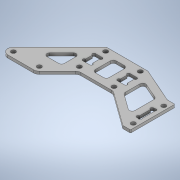
# Autodesk Inventor part: Head_side_frame_
Saved by Autodesk Inventor 2020.4 (Build 244396000, 396)
## iProperties
Created: 2022-01-01
Part Number: Head_side_frame_
Material: GFRP
Document SubType Name: Modeling
Designer: Masato Kubotera
Density: 1.75 g/cm^3
Appearance: 滑らか - 標準の灰色
Description: GFRP T2
Mass: 6.0022 g
Surface Area: 45.99 cm^2
Volume: 3.42983 cm^3
Author: Masato Kubotera
Autodesk Inventor part; units mm, degrees
ref_plane "YZ Plane" through (0, 0, 0) normal (1, 0, 0) x (0, 1, 0)
ref_plane "XZ Plane" through (0, 0, 0) normal (0, 1, 0) x (-1, 0, 0)
ref_plane "XY Plane" through (0, 0, 0) normal (0, 0, 1) x (1, 0, 0)
derived "Head_basis.ipt"
sketch "スケッチ1" plane through (0, 0, 0) normal (0, 1, 0) x (-1, 0, 0)
  line L0 (-44.985, 63.28) -> (-70.7944, 37.4706) construction
  line L1 (5.295, 20.5) -> (-9.705, 20.5)
  line L2 (-2.205, 20.5) -> (-44.985, 63.28) construction
  line L3 (-2.205, 20.5) -> (-2.205, 4.9887) construction
  line L4 (-54.1774, 43.481) -> (-57.7129, 47.0165) construction
  line L5 (-57.7129, 47.0165) -> (-80.3403, 24.3891) construction
  line L6 (-80.3403, 24.3891) -> (-76.8048, 20.8536) construction
  line L7 (-76.8048, 20.8536) -> (-54.1774, 43.481) construction
  line L8 (-54.1774, 43.481) -> (-80.3403, 24.3891) construction
  line L9 (-57.7129, 47.0165) -> (-76.8048, 20.8536) construction
  line L10 (-61.9555, 39.2383) -> (-72.5621, 28.6317) construction
  line L11 (-70.7944, 26.864) -> (-60.1878, 37.4706) construction
  circle A0 centre (-59.4807, 41.7132) radius 1.6
  line L12 (-55.9451, 45.2487) -> (-78.5725, 22.6213) construction
  line L13 (7.845, -2.5) -> (7.845, 2.5) construction
  line L14 (17.795, -2.5) -> (-22.205, -2.5) construction
  line L15 (6.3601, -2.5) -> (6.3601, 2.5) construction
  line L16 (7.795, -2.5) -> (7.795, 2.5)
  line L17 (11.414, 2.5) -> (7.545, 2.5)
  line L18 (-12.205, -2.5) -> (-12.205, 2.5)
  line L19 (5.6411, 2.5) -> (7.6411, 2.5)
  line L20 (-17.705, 0.5) -> (-15.205, 0.5)
  line L21 (7.795, 2.5) -> (-12.205, 2.5)
  line L22 (-15.205, 2.5) -> (10.795, 2.5) construction
  line L23 (-24.705, -2.5) -> (20.295, -2.5)
  arc A1 (7.795, -2.5) -> (9.895, -2.5) centre (8.845, -2.5) ccw
  line L24 (9.795, -2.5) -> (11.795, -2.5)
  line L25 (9.795, -2.5) -> (22.795, -2.5)
  line L26 (22.795, -2.5) -> (22.795, -5.5)
  line L27 (22.795, -5.5) -> (14.045, -5.5)
  line L28 (17.795, -2.5) -> (17.795, -5.5) construction
  arc A2 (-14.305, -2.5) -> (-12.205, -2.5) centre (-13.255, -2.5) ccw
  line L29 (-14.205, -2.5) -> (-27.205, -2.5)
  line L30 (-27.205, -2.5) -> (-27.205, -5.5)
  line L31 (-22.205, -2.5) -> (-22.205, -5.5) construction
  line L32 (-18.455, -5.5) -> (-27.205, -5.5)
  circle A3 centre (-11.5482, -8.5) radius 2
  arc A4 (14.045, -5.5) -> (11.1379, -8.4177) centre (14.045, -8.4071) ccw
  line L33 (15.045, -5.5) -> (15.045, -6.9) construction
  line L34 (15.045, -6.9) -> (20.545, -6.9) construction
  line L35 (20.545, -5.5) -> (20.545, -6.9) construction
  circle A5 centre (-11.5482, -8.5) radius 4
  line L36 (22.795, -2.5) -> (22.795, 0.5)
  line L37 (-2.205, -12.0113) -> (-2.205, 4.9887) construction
  line L38 (-19.455, -5.5) -> (-19.455, -6.9) construction
  line L39 (-19.455, -6.9) -> (-24.955, -6.9) construction
  line L40 (-24.955, -5.5) -> (-24.955, -6.9) construction
  line L41 (-69.0266, 35.7028) -> (-65.4911, 32.1673) construction
  circle A6 centre (-75.037, 26.1569) radius 1.6
  line L42 (-32.205, -2.5) -> (-22.205, -2.5)
  circle A7 centre (1.665, -21.7132) radius 2
  arc A8 (4.4934, -24.5416) -> (11.1379, -8.4177) centre (-11.5482, -8.5) ccw
  line L43 (-14.3767, -11.3284) -> (-1.1635, -24.5416)
  circle A9 centre (1.665, -21.7132) radius 4
  line L44 (4.4934, -18.8848) -> (-8.7198, -5.6716)
  line L45 (1.665, -21.7132) -> (-11.5482, -8.5) construction
  line L46 (-49.2969, -22.1777) -> (-31.6192, -4.5) construction
  line L47 (-31.6192, -4.5) -> (-28.0837, -8.0355) construction
  line L48 (-28.0837, -8.0355) -> (-45.7614, -25.7132) construction
  line L49 (-45.7614, -25.7132) -> (-49.2969, -22.1777) construction
  line L50 (-49.2969, -22.1777) -> (-28.0837, -8.0355) construction
  line L51 (-31.6192, -4.5) -> (-45.7614, -25.7132) construction
  line L52 (-47.5291, -23.9454) -> (-29.8515, -6.2678) construction
  line L53 (-40.4581, -13.3388) -> (-36.9225, -16.8744) construction
  line L54 (-40.1045, -20.0563) -> (-33.7405, -13.6924) construction
  line L55 (-33.7405, -13.6924) -> (-37.2761, -10.1569) construction
  line L56 (-37.2761, -10.1569) -> (-43.64, -16.5208) construction
  line L57 (-43.64, -16.5208) -> (-40.1045, -20.0563) construction
  line L58 (-40.1045, -20.0563) -> (-37.2761, -10.1569) construction
  line L59 (-33.7405, -13.6924) -> (-43.64, -16.5208) construction
  circle A10 centre (-45.4078, -21.8241) radius 1.6
  line L60 (-42.2258, -15.0359) -> (-38.761, -11.5711)
  line L61 (-37.2761, -10.0861) -> (-33.6698, -13.6924)
  line L62 (-35.1548, -15.1773) -> (-38.6196, -18.6421)
  line L63 (-40.1045, -20.1271) -> (-43.7107, -16.5208)
  line L64 (-43.7107, -16.5208) -> (-33.6698, -13.6924) construction
  line L65 (-37.2761, -10.0861) -> (-40.1045, -20.1271) construction
  arc A11 (-42.2258, -15.0359) -> (-43.7107, -16.5208) centre (-42.9683, -15.7784) ccw
  arc A12 (-37.2761, -10.0861) -> (-38.761, -11.5711) centre (-38.0185, -10.8286) ccw
  circle A13 centre (-31.9728, -8.3891) radius 1.6
  line L66 (-41.8723, -18.2886) -> (-35.5083, -11.9246) construction
  arc A14 (-40.1045, -20.1271) -> (-38.6196, -18.6421) centre (-39.362, -19.3846) ccw
  arc A15 (-35.1548, -15.1773) -> (-33.6698, -13.6924) centre (-34.4123, -14.4349) ccw
  line L67 (-32.205, 14.5) -> (-24.205, 22.5)
  circle A16 centre (-32.205, -2.5) radius 1 construction
  line L68 (-11.5482, -4.5) -> (-31.6192, -4.5)
  line L69 (-58.0664, 47.3701) -> (-54.1774, 43.481)
  line L70 (-76.8048, 20.8536) -> (-80.6939, 24.7426)
  line L71 (-80.6939, 24.7426) -> (-58.0664, 47.3701)
  line L72 (-45.7614, -25.7132) -> (1.665, -25.7132)
  line L73 (-45.7614, -25.7132) -> (-49.2969, -22.1777)
  arc A17 (-15.5479, -8.4464) -> (-18.455, -5.5) centre (-18.455, -8.4074) ccw
  line L74 (-49.2969, 13.1777) -> (-45.7614, 9.6421) construction
  line L75 (-45.7614, 9.6421) -> (-63.439, -8.0355) construction
  line L76 (-49.2969, 13.1777) -> (-63.439, -8.0355) construction
  arc A18 (-59.9035, 2.6418) -> (-61.3884, 1.1569) centre (-60.646, 1.8993) ccw
  line L77 (-52.8324, 2.5004) -> (-56.2972, -0.9645)
  line L78 (-57.7822, -2.4494) -> (-61.3884, 1.1569)
  line L79 (-61.3177, 1.1569) -> (-57.7822, -2.3787) construction
  line L80 (-66.9746, -4.5) -> (-49.2969, 13.1777) construction
  line L81 (-58.1357, 4.3388) -> (-54.6002, 0.8033) construction
  arc A19 (-57.7822, -2.4494) -> (-56.2972, -0.9645) centre (-57.0397, -1.7069) ccw
  line L82 (-59.5499, -0.6109) -> (-53.186, 5.753) construction
  line L83 (-59.9035, 2.6418) -> (-56.4387, 6.1066)
  line L84 (-51.4182, 3.9853) -> (-61.3177, 1.1569) construction
  line L85 (-61.3884, 1.1569) -> (-51.3475, 3.9853) construction
  arc A20 (-52.8324, 2.5004) -> (-51.3475, 3.9853) centre (-52.09, 3.2428) ccw
  line L86 (-57.7822, -2.3787) -> (-51.4182, 3.9853) construction
  line L87 (-54.9537, 7.5208) -> (-61.3177, 1.1569) construction
  arc A21 (-54.9537, 7.5915) -> (-56.4387, 6.1066) centre (-55.6962, 6.8491) ccw
  line L88 (-57.7822, -2.3787) -> (-54.9537, 7.5208) construction
  line L89 (-51.4182, 3.9853) -> (-54.9537, 7.5208) construction
  line L90 (-54.9537, 7.5915) -> (-51.3475, 3.9853)
  circle A22 centre (-49.6504, 9.2886) radius 1.6
  line L91 (-66.9746, -4.5) -> (-45.7614, 9.6421) construction
  line L92 (-65.2068, -6.2678) -> (-47.5291, 11.4099) construction
  line L93 (-54.9537, 7.5915) -> (-57.7822, -2.4494) construction
  line L94 (-63.439, -8.0355) -> (-66.9746, -4.5) construction
  circle A23 centre (-63.0855, -4.1464) radius 1.6
  line L95 (-63.439, -8.0355) -> (-66.9746, -4.5)
  line L96 (-31.6192, -4.5) -> (-45.7614, 9.6421)
  line L97 (-49.2969, 13.1777) -> (-45.7614, 9.6421)
  line L98 (-49.2969, 13.1777) -> (-54.1774, 43.481)
  line L99 (-76.8048, 20.8536) -> (-66.9746, -4.5)
  line L100 (-63.439, -8.0355) -> (-49.2969, -22.1777)
  line L101 (-54.1774, 43.481) -> (-76.8048, 20.8536) construction
  line L102 (-56.9363, 29.166) -> (-54.8022, 15.9153)
  line L103 (-55.3626, 14.1831) -> (-62.9161, 6.6295)
  line L104 (-66.1951, 7.3207) -> (-70.4935, 18.407)
  line L105 (-70.043, 20.5443) -> (-60.3251, 30.2622)
  arc A24 (-56.9363, 29.166) -> (-60.3251, 30.2622) centre (-58.9109, 28.848) ccw
  arc A25 (-70.043, 20.5443) -> (-70.4935, 18.407) centre (-68.6288, 19.13) ccw
  arc A26 (-66.1951, 7.3207) -> (-62.9161, 6.6295) centre (-64.3303, 8.0437) ccw
  arc A27 (-55.3626, 14.1831) -> (-54.8022, 15.9153) centre (-56.7768, 15.5973) ccw
  line L106 (-15.4772, -17.299) -> (-21.4624, -11.3138)
  line L107 (-24.2908, -11.3138) -> (-30.2761, -17.299)
  line L108 (-28.8619, -20.7132) -> (-16.8914, -20.7132)
  arc A28 (-16.8914, -20.7132) -> (-15.4772, -17.299) centre (-16.8914, -18.7132) ccw
  arc A29 (-21.4624, -11.3138) -> (-24.2908, -11.3138) centre (-22.8766, -12.728) ccw
  arc A30 (-30.2761, -17.299) -> (-28.8619, -20.7132) centre (-28.8619, -18.7132) ccw
  line L109 (-40.1045, -3.0858) -> (-44.3471, 1.1569)
  line L110 (-47.1756, 1.1569) -> (-54.9537, -6.6213)
  line L111 (-54.9537, -9.4497) -> (-50.7111, -13.6924)
  line L112 (-47.8827, -13.6924) -> (-40.1045, -5.9142)
  arc A31 (-40.1045, -5.9142) -> (-40.1045, -3.0858) centre (-41.5187, -4.5) ccw
  arc A32 (-44.3471, 1.1569) -> (-47.1756, 1.1569) centre (-45.7614, -0.2574) ccw
  arc A33 (-54.9537, -6.6213) -> (-54.9537, -9.4497) centre (-53.5395, -8.0355) ccw
  arc A34 (-50.7111, -13.6924) -> (-47.8827, -13.6924) centre (-49.2969, -12.2782) ccw
  circle A35 centre (-11.5482, -8.5) radius 1.6
  circle A36 centre (1.665, -21.7132) radius 1.6
  line L113 (-61.2484, 36.4099) -> (-69.7337, 27.9246) construction
  line L114 (-69.7337, 27.9246) -> (-71.5015, 29.6924) construction
  line L115 (-71.5015, 29.6924) -> (-63.0162, 38.1777) construction
  line L116 (-63.0162, 38.1777) -> (-61.2484, 36.4099) construction
  line L117 (-61.2484, 36.4099) -> (-71.5015, 29.6924) construction
  line L118 (-69.7337, 27.9246) -> (-63.0162, 38.1777) construction
  line L119 (-62.1323, 37.2938) -> (-70.6176, 28.8085) construction
  line L120 (-61.1777, 36.4099) -> (-63.0162, 38.2484)
  line L121 (-63.0162, 38.2484) -> (-71.5722, 29.6924)
  line L122 (-71.5722, 29.6924) -> (-69.7337, 27.8539)
  line L123 (-69.7337, 27.8539) -> (-61.1777, 36.4099)
  line L124 (-61.1777, 36.4099) -> (-71.5722, 29.6924) construction
  line L125 (-63.0162, 38.2484) -> (-69.7337, 27.8539) construction
  arc A37 (-62.6626, 34.925) -> (-61.1777, 36.4099) centre (-61.9202, 35.6674) ccw
  arc A38 (-61.9662, 37.1984) -> (-64.0662, 37.1984) centre (-63.0162, 37.1984) ccw
  arc A39 (-69.7337, 27.8539) -> (-68.2488, 29.3388) centre (-68.9912, 28.5964) ccw
  arc A40 (-70.5222, 30.7424) -> (-70.5222, 28.6424) centre (-70.5222, 29.6924) ccw
  point P0 (0, 0)
  point P1 (-67.2588, 33.935)
  point P2 (7.6045, 2.5)
  point P3 (-38.6903, -15.1066)
  point P4 (-38.6903, -15.1066)
  point P5 (-56.368, 2.5711)
  point P6 (-56.368, 2.5711)
  point P7 (-54.6397, 14.906)
  point P8 (-66.3749, 33.0511)
  point P9 (-66.3749, 33.0511)
  point P10 (-70.5222, 28.6424)
  point P11 (-70.5222, 30.7424)
  point P12 (-68.2488, 29.3388)
  dimension "d5" = 0.5
  measures "d5" distance between parallel lines of L71 L5
extrude "押し出し1" add sketch "スケッチ1" along normal blind 2 contours L68 A5 A17 L32 L30 | L30 L32 A17 A5 L43 A9 L72 L73 L100 L95 L99 L70 L71 L69 L98 L97 L96 L68 | A5 | L44 A9 L43 A5 | A9 | A3 | A7
fillet "フィレット1" radius 4 3 edges at (31.6192, 1, -4.5) (49.2969, 1, 13.1777) (76.8048, 1, 20.8536)
fillet "フィレット2" radius 0.5 2 edges at (58.0664, 1, 47.3701) (80.6939, 1, 24.7426)
equation "\"d4\" = d5"
